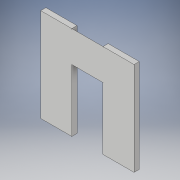
# Autodesk Inventor part: BackLiftProtoPart3
Saved by Autodesk Inventor 2017 (Build 210142000, 142)
## iProperties
Created: 2017-11-11
Part Number: BackLiftProtoPart3
Material: Generic
Document SubType Name: Modeling
Designer: User
Density: 1 g/cm^3
Appearance: Default
Author: User
Autodesk Inventor part; units mm, degrees
ref_plane "YZ Plane" through (0, 0, 0) normal (1, 0, 0) x (0, 1, 0)
ref_plane "XZ Plane" through (0, 0, 0) normal (0, 1, 0) x (-1, 0, 0)
ref_plane "XY Plane" through (0, 0, 0) normal (0, 0, 1) x (1, 0, 0)
sketch "Sketch1" plane through (0, 0, 0) normal (0, 0, 1) x (1, 0, 0)
  line L0 (0, 0) -> (457.2, 0)
  line L1 (457.2, 0) -> (457.2, 457.2)
  line L2 (457.2, 457.2) -> (0, 457.2)
  line L3 (0, 457.2) -> (0, 0)
  dimension "d0" = 457.2
  dimension "d1" = 457.2
  constraints: 8 end point, 2 parallel, 1 horizontal, 1 perpendicular
  measures "d0" distance of L2.end L1.end
  measures "d1" distance of L1.end L0.end
extrude "Extrusion1" add sketch "Sketch1" along normal blind 25.4
sketch "Sketch2" plane through (0, 0, 0) normal (-1, 0, 0) x (0, 0, 1)
  line L0 (0, 457.2) -> (25.4, 457.2) projected
  line L1 (0, 457.2) -> (0, 304.8)
  line L2 (0, 0) -> (0, 457.2) projected
  line L3 (25.4, 0) -> (25.4, 457.2) projected
  line L4 (0, 304.8) -> (25.4, 457.2)
  dimension "d4" = 152.4
  constraints: 4 end point, 1 point on line
  measures "d4" distance of L0.start L1.end
extrude "Extrusion2" cut sketch "Sketch2" against normal blind 457.2
sketch "Sketch3" plane through (0, 0, 0) normal (-1, 0, 0) x (0, 0, 1)
  line L0 (25.4, 457.2) -> (25.4, 0) projected
  line L1 (25.4, 457.2) -> (0, 457.2)
  line L2 (0, 304.8) -> (0, 0) projected
  line L3 (0, 457.2) -> (0, 304.8)
  line L4 (0, 304.8) -> (25.4, 457.2)
  constraints: 6 end point, 1 horizontal, 1 perpendicular
extrude "Extrusion3" add sketch "Sketch3" against normal blind 152.4
sketch "Sketch4" plane through (457.2, 0, 25.4) normal (1, 0, 0) x (0, 0, -1)
  line L0 (0, 0) -> (0, 457.2) projected
  line L1 (0, 457.2) -> (25.4, 457.2)
  line L2 (25.4, 304.8) -> (0, 457.2) projected
  line L3 (25.4, 457.2) -> (25.4, 304.8)
  line L4 (25.4, 304.8) -> (0, 457.2)
  point P0 (25.4, 0)
  constraints: 6 end point, 1 collinear, 1 horizontal, 1 perpendicular
extrude "Extrusion4" add sketch "Sketch4" against normal blind 152.4
sketch "Sketch5" plane through (0, 0, 0) normal (0, -1, 0) x (1, 0, 0)
  line L0 (304.8, 25.4) -> (152.4, 25.4) projected
  line L1 (304.8, 25.4) -> (152.4, 25.4)
  line L2 (152.4, 25.4) -> (152.4, 0)
  line L3 (152.4, 0) -> (304.8, 0)
  line L4 (304.8, 0) -> (304.8, 25.4)
  point P0 (0, 0)
  constraints: 8 end point, 2 parallel, 1 horizontal, 1 perpendicular
extrude "Extrusion5" cut sketch "Sketch5" against normal blind 304.8
body "Solid1"
